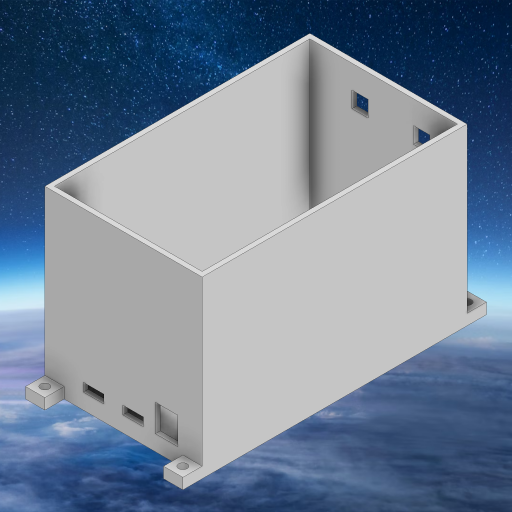
# Autodesk Inventor part: base
Saved by Autodesk Inventor 2023 (Build 270158000, 158)
## iProperties
Created: 2023-09-17
Part Number: base
Material: 一般
Document SubType Name: Modeling
Designer: 310611102
Density: 1 g/cm^3
Appearance: 預設
Author: 310611102
Autodesk Inventor part; units mm, degrees
ref_plane "YZ Plane" through (0, 0, 0) normal (1, 0, 0) x (0, 1, 0)
ref_plane "XZ Plane" through (0, 0, 0) normal (0, 1, 0) x (-1, 0, 0)
ref_plane "XY Plane" through (0, 0, 0) normal (0, 0, 1) x (1, 0, 0)
sketch "Sketch1" plane through (0, 0, 0) normal (0, 1, 0) x (-1, 0, 0)
  line L0 (32.65, 55) -> (-32.65, 55)
  line L1 (-32.65, 55) -> (-32.65, -55)
  line L2 (-32.65, -55) -> (32.65, -55)
  line L3 (32.65, -55) -> (32.65, 55)
  line L4 (32.65, 55) -> (-32.65, -55) construction
  line L5 (-32.65, 55) -> (32.65, -55) construction
  circle A0 centre (-24.15, 38) radius 1.75
  circle A1 centre (-24.15, -45) radius 1.75
  circle A2 centre (24.15, 37) radius 1.75
  circle A3 centre (24.15, -38) radius 1.75
  point P0 (0, 0)
  dimension "d0" = 110
  dimension "d1" = 65.3
  dimension "d2" = 83
  dimension "d3" = 8.5
  dimension "d4" = 17
  dimension "d5" = 3.5
  dimension "d6" = 3.5
  dimension "d7" = 3.5
  dimension "d8" = 1
  dimension "d9" = 48.3
  dimension "d10" = 3.5
  dimension "d11" = 75
  constraints: 12 end point, 4 centre point, 2 midpoint, 2 parallel, 2 vertical alignment, 1 horizontal, 1 perpendicular
  measures "d0" distance of L0.end L1.end
  measures "d1" distance of L1.end L2.end
  measures "d2" distance of A1.centre A0.centre
  measures "d3" distance from line of L1 A1.centre
  measures "d4" distance from line of L0 A0.centre
  measures "d5" diameter of A0
  measures "d6" diameter of A1
  measures "d7" diameter of A2
  measures "d8" vertical distance of A0.centre A2.centre
  measures "d9" horizontal distance of A0.centre A2.centre
  measures "d10" diameter of A3
  measures "d11" distance of A3.centre A2.centre
extrude "Extrusion1" add sketch "Sketch1" along normal blind 2
sketch "Sketch2" plane through (-32.65, 0, 55) normal (0, 0, 1) x (1, 0, 0)
  line L0 (0, 70) -> (65.3, 70)
  line L1 (65.3, 70) -> (65.3, 0)
  line L2 (65.3, 0) -> (0, 0)
  line L3 (0, 0) -> (0, 70)
  line L4 (0, 70) -> (65.3, 0) construction
  line L5 (65.3, 70) -> (0, 0) construction
  line L6 (65.3, 0) -> (65.3, 2) projected
  line L7 (16, 7.5) -> (24.5, 7.5)
  line L8 (24.5, 7.5) -> (24.5, 4)
  line L9 (24.5, 4) -> (16, 4)
  line L10 (16, 4) -> (16, 7.5)
  line L11 (16, 7.5) -> (24.5, 4) construction
  line L12 (24.5, 7.5) -> (16, 4) construction
  line L13 (32.4, 7.5) -> (40.9, 7.5)
  line L14 (40.9, 7.5) -> (40.9, 4)
  line L15 (40.9, 4) -> (32.4, 4)
  line L16 (32.4, 4) -> (32.4, 7.5)
  line L17 (32.4, 7.5) -> (40.9, 4) construction
  line L18 (40.9, 7.5) -> (32.4, 4) construction
  line L19 (45.9, 15.3) -> (55.2, 15.3)
  line L20 (55.2, 15.3) -> (55.2, 4)
  line L21 (55.2, 4) -> (45.9, 4)
  line L22 (45.9, 4) -> (45.9, 15.3)
  line L23 (45.9, 15.3) -> (55.2, 4) construction
  line L24 (55.2, 15.3) -> (45.9, 4) construction
  line L25 (0, 2) -> (65.3, 2) projected
  point P0 (32.65, 0)
  point P1 (32.65, 35)
  point P2 (20.25, 5.75)
  point P3 (36.65, 5.75)
  point P4 (50.55, 9.65)
  point P5 (45.9, 9.65)
  dimension "d14" = 70
  dimension "d15" = 11.3
  dimension "d16" = 9.3
  dimension "d17" = 8.5
  dimension "d18" = 3.5
  dimension "d19" = 8.5
  dimension "d20" = 3.5
  dimension "d21" = 2
  dimension "d22" = 7.9
  dimension "d23" = 16
  dimension "d24" = 5
  constraints: 48 end point, 9 midpoint, 8 parallel, 4 horizontal, 4 perpendicular, 2 point on line, 1 collinear
  measures "d14" distance of L0.end L1.end
  measures "d15" distance of L19.end L20.end
  measures "d16" distance of L19.start L19.end
  measures "d17" distance of L7.start L7.end
  measures "d18" distance of L9.end L7.start
  measures "d19" distance of L13.start L13.end
  measures "d20" distance of L15.end L13.start
  measures "d21" distance between parallel lines of L25 L9
  measures "d22" distance between parallel lines of L16 L8
  measures "d23" distance between parallel lines of L3 L10
  measures "d24" distance from line of point (45.9, 9.65) L14
extrude "Extrusion2" add sketch "Sketch2" against normal blind 2 contours L0 L1 L25 L3
sketch "Sketch3" plane through (32.65, 0, 55) normal (1, 0, 0) x (0, 0, -1)
  line L0 (110, 0) -> (110, 2) projected
  line L1 (0, 70) -> (110, 70)
  line L2 (110, 70) -> (110, 0)
  line L3 (110, 0) -> (0, 0)
  line L4 (0, 0) -> (0, 70)
  line L5 (0, 70) -> (110, 0) construction
  line L6 (110, 70) -> (0, 0) construction
  point P0 (55, 0)
  point P1 (55, 35)
  point P2 (0, 70)
  constraints: 12 end point, 2 midpoint, 2 parallel, 1 coincident, 1 horizontal, 1 perpendicular
extrude "Extrusion3" add sketch "Sketch3" against normal blind 2
sketch "Sketch4" plane through (-32.65, 0, -55) normal (-1, 0, 0) x (0, 0, 1)
  line L0 (110, 0) -> (110, 70) projected
  line L1 (0, 70) -> (110, 70)
  line L2 (110, 70) -> (110, 0)
  line L3 (110, 0) -> (0, 0)
  line L4 (0, 0) -> (0, 70)
  line L5 (0, 70) -> (110, 0) construction
  line L6 (110, 70) -> (0, 0) construction
  point P0 (55, 0)
  point P1 (55, 35)
  point P2 (0, 70)
  constraints: 12 end point, 2 midpoint, 2 parallel, 1 coincident, 1 horizontal, 1 perpendicular
extrude "Extrusion4" add sketch "Sketch4" against normal blind 2
sketch "Sketch5" plane through (32.65, 0, -55) normal (0, 0, -1) x (-1, 0, 0)
  line L0 (65.3, 0) -> (65.3, 70) projected
  line L1 (0, 70) -> (65.3, 70)
  line L2 (65.3, 70) -> (65.3, 0)
  line L3 (65.3, 0) -> (0, 0)
  line L4 (0, 0) -> (0, 70)
  line L5 (0, 70) -> (65.3, 0) construction
  line L6 (65.3, 70) -> (0, 0) construction
  line L7 (13.5, 60.35) -> (20.2, 60.35)
  line L8 (20.2, 60.35) -> (20.2, 53.65)
  line L9 (20.2, 53.65) -> (13.5, 53.65)
  line L10 (13.5, 53.65) -> (13.5, 60.35)
  line L11 (13.5, 60.35) -> (20.2, 53.65) construction
  line L12 (20.2, 60.35) -> (13.5, 53.65) construction
  line L13 (39.1, 60.35) -> (45.8, 60.35)
  line L14 (45.8, 60.35) -> (45.8, 53.65)
  line L15 (45.8, 53.65) -> (39.1, 53.65)
  line L16 (39.1, 53.65) -> (39.1, 60.35)
  line L17 (39.1, 60.35) -> (45.8, 53.65) construction
  line L18 (45.8, 60.35) -> (39.1, 53.65) construction
  line L19 (2, 2) -> (63.3, 2) projected
  point P0 (32.65, 0)
  point P1 (32.65, 35)
  point P2 (16.85, 57)
  point P3 (42.45, 57)
  point P4 (20.2, 57)
  point P5 (39.1, 57)
  point P6 (45.8, 57)
  dimension "d31" = 6.7
  dimension "d32" = 6.7
  dimension "d33" = 6.7
  dimension "d34" = 6.7
  dimension "d35" = 18.9
  dimension "d36" = 13.5
  dimension "d38" = 55
  dimension "d39" = 19.5
  constraints: 36 end point, 9 midpoint, 6 parallel, 3 horizontal, 3 perpendicular, 1 coincident, 1 horizontal alignment
  measures "d31" distance of L8.end L9.end
  measures "d32" distance of L7.end L8.end
  measures "d33" distance of L14.end L15.end
  measures "d34" distance of L13.end L14.end
  measures "d35" distance of point (20.2, 57) point (39.1, 57)
  measures "d36" distance between parallel lines of L4 L10
  measures "d38" distance from line of L19 point (16.85, 57)
  measures "d39" distance from line of L0 point (45.8, 57)
extrude "Extrusion5" add sketch "Sketch5" against normal blind 2
sketch "Sketch6" plane through (0, 0, 0) normal (0, -1, 0) x (1, 0, 0)
  line L0 (-32.65, -55) -> (32.65, -55) projected
  line L1 (-24.65, -63) -> (-32.65, -63)
  line L2 (-32.65, -63) -> (-32.65, -55)
  line L3 (-32.65, -55) -> (-24.65, -55)
  line L4 (-24.65, -55) -> (-24.65, -63)
  line L5 (-24.65, -63) -> (-32.65, -55) construction
  line L6 (-32.65, -63) -> (-24.65, -55) construction
  line L7 (0, 0) -> (-42.6536, 0) construction
  line L8 (0, 0) -> (0, 77.6951) construction
  line L9 (-24.65, 63) -> (-32.65, 63)
  line L10 (-32.65, 63) -> (-32.65, 55)
  line L11 (-32.65, 55) -> (-24.65, 55)
  line L12 (-24.65, 55) -> (-24.65, 63)
  line L13 (-24.65, 63) -> (-32.65, 55) construction
  line L14 (-32.65, 63) -> (-24.65, 55) construction
  line L15 (24.65, -63) -> (32.65, -63)
  line L16 (32.65, -63) -> (32.65, -55)
  line L17 (32.65, -55) -> (24.65, -55)
  line L18 (24.65, -55) -> (24.65, -63)
  line L19 (24.65, -63) -> (32.65, -55) construction
  line L20 (32.65, -63) -> (24.65, -55) construction
  line L21 (24.65, 63) -> (32.65, 63)
  line L22 (32.65, 63) -> (32.65, 55)
  line L23 (32.65, 55) -> (24.65, 55)
  line L24 (24.65, 55) -> (24.65, 63)
  line L25 (24.65, 63) -> (32.65, 55) construction
  line L26 (32.65, 63) -> (24.65, 55) construction
  circle A0 centre (-28.65, -59) radius 1.75
  circle A1 centre (-28.65, 59) radius 1.75
  circle A2 centre (28.65, -59) radius 1.75
  circle A3 centre (28.65, 59) radius 1.75
  point P0 (-28.65, 59)
  point P1 (28.65, 59)
  dimension "d42" = 8
  dimension "d43" = 8
  dimension "d44" = 3.5
  constraints: 52 end point, 17 symmetric about line, 4 centre point, 2 horizontal, 2 midpoint, 2 parallel, 1 coincident, 1 perpendicular, 1 vertical, 3 other
  measures "d42" distance of L1.start L1.end
  measures "d43" distance of L1.end L0.start
  measures "d44" diameter of A0
extrude "Extrusion6" add sketch "Sketch6" against normal blind 2
sketch "Sketch7" plane through (0, 0, 0) normal (0, -1, 0) x (1, 0, 0)
  circle A0 centre (-24.15, -38) radius 1.75 projected
  line L0 (-24.15, -34.6514) -> (-21.25, -36.3257)
  line L1 (-21.25, -36.3257) -> (-21.25, -39.6743)
  line L2 (-21.25, -39.6743) -> (-24.15, -41.3486)
  line L3 (-24.15, -41.3486) -> (-27.05, -39.6743)
  line L4 (-27.05, -39.6743) -> (-27.05, -36.3257)
  line L5 (-27.05, -36.3257) -> (-24.15, -34.6514)
  circle A1 centre (-24.15, 37) radius 1.75 projected
  line L6 (-24.15, 40.3486) -> (-21.25, 38.6743)
  line L7 (-21.25, 38.6743) -> (-21.25, 35.3257)
  line L8 (-21.25, 35.3257) -> (-24.15, 33.6514)
  line L9 (-24.15, 33.6514) -> (-27.05, 35.3257)
  line L10 (-27.05, 35.3257) -> (-27.05, 38.6743)
  line L11 (-27.05, 38.6743) -> (-24.15, 40.3486)
  circle A2 centre (24.15, 38) radius 1.75 projected
  line L12 (24.15, 41.3486) -> (27.05, 39.6743)
  line L13 (27.05, 39.6743) -> (27.05, 36.3257)
  line L14 (27.05, 36.3257) -> (24.15, 34.6514)
  line L15 (24.15, 34.6514) -> (21.25, 36.3257)
  line L16 (21.25, 36.3257) -> (21.25, 39.6743)
  line L17 (21.25, 39.6743) -> (24.15, 41.3486)
  circle A3 centre (24.15, -45) radius 1.75 projected
  line L18 (24.15, -41.6514) -> (27.05, -43.3257)
  line L19 (27.05, -43.3257) -> (27.05, -46.6743)
  line L20 (27.05, -46.6743) -> (24.15, -48.3486)
  line L21 (24.15, -48.3486) -> (21.25, -46.6743)
  line L22 (21.25, -46.6743) -> (21.25, -43.3257)
  line L23 (21.25, -43.3257) -> (24.15, -41.6514)
  circle A4 centre (-28.65, 59) radius 1.75 projected
  circle A5 centre (28.65, -59) radius 1.75 projected
  circle A6 centre (28.65, 59) radius 1.75 projected
  circle A7 centre (-28.65, -59) radius 1.75 projected
  circle A8 centre (-24.15, -38) radius 1.75 projected
  circle A9 centre (-24.15, 37) radius 1.75 projected
  circle A10 centre (24.15, -45) radius 1.75 projected
  circle A11 centre (24.15, 38) radius 1.75 projected
  line L24 (32.65, 63) -> (32.65, -63) projected
  line L25 (32.65, 63) -> (24.65, 63) projected
  line L26 (24.65, 63) -> (24.65, 55) projected
  line L27 (-24.65, 55) -> (24.65, 55) projected
  line L28 (-24.65, 55) -> (-24.65, 63) projected
  line L29 (-24.65, 63) -> (-32.65, 63) projected
  line L30 (-32.65, 63) -> (-32.65, -63) projected
  line L31 (-32.65, -63) -> (-24.65, -63) projected
  line L32 (-24.65, -63) -> (-24.65, -55) projected
  line L33 (24.65, -55) -> (-24.65, -55) projected
  line L34 (24.65, -55) -> (24.65, -63) projected
  line L35 (24.65, -63) -> (32.65, -63) projected
  point P0 (0, 0)
  point P1 (27.05, 38)
  point P2 (21.25, 38)
  point P3 (27.05, -45)
  point P4 (21.25, -45)
  dimension "d47" = 5.8
  dimension "d48" = 5.8
  dimension "d49" = 5.8
  dimension "d50" = 5.8
  constraints: 48 end point, 4 coincident, 4 midpoint, 52 other
  measures "d47" distance between parallel lines of L1 L4
  measures "d48" distance between parallel lines of L7 L10
  measures "d49" distance of point (27.05, 38) point (21.25, 38)
  measures "d50" distance of point (27.05, -45) point (21.25, -45)
extrude "Extrusion7" add sketch "Sketch7" along normal blind 2.5 contours L24 L35 L34 L33 L32 L31 L30 L29 L28 L27 L26 L25
equation "\"d6\" = d5"
equation "\"d7\" = d5"
equation "\"d10\" = d5"
equation "\"d48\" = d47"
equation "\"d49\" = d47"
equation "\"d50\" = d47"
body "Solid1"
